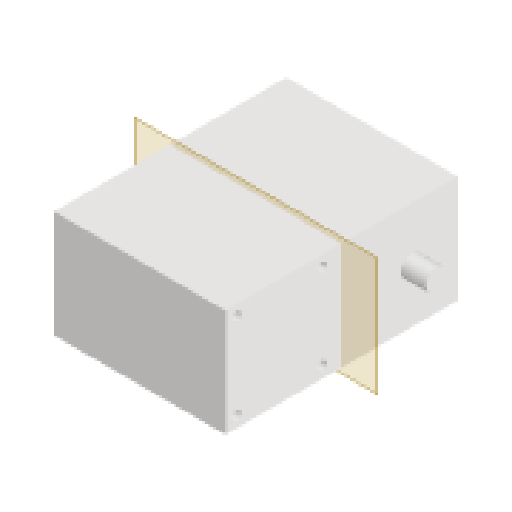
# Autodesk Inventor part: рдс150
Saved by Autodesk Inventor 2023.2 (Build 272271030, 271C)
## iProperties
Created: 2025-05-06
Part Number: рдс150
Material: Типовые
Document SubType Name: Modeling
Designer: Олег Коноваленко
Density: 1 g/cm^3
Appearance: По умолчанию
Author: Олег Коноваленко
Autodesk Inventor part; units mm, degrees
ref_plane "YZ Plane" through (0, 0, 0) normal (1, 0, 0) x (0, 1, 0)
ref_plane "XZ Plane" through (0, 0, 0) normal (0, 1, 0) x (-1, 0, 0)
ref_plane "XY Plane" through (0, 0, 0) normal (0, 0, 1) x (1, 0, 0)
sketch "Эскиз1" plane through (0, 0, 0) normal (0, 1, 0) x (-1, 0, 0)
  line L0 (24, -32.5) -> (-24, -32.5)
  line L1 (-24, -32.5) -> (-24, 32.5)
  line L2 (-24, 32.5) -> (24, 32.5)
  line L3 (24, 32.5) -> (24, -32.5)
  line L4 (24, -32.5) -> (-24, 32.5) construction
  line L5 (-24, -32.5) -> (24, 32.5) construction
  line L6 (-33.6, 0) -> (33.6, 0) construction
  line L7 (0, -45.5) -> (0, 45.5) projected
  point P0 (0, 0)
  point P1 (0, 0)
  point P2 (0, 0)
  dimension "d0" = 65
  dimension "d1" = 48
  constraints: 12 end point, 4 midpoint, 2 parallel, 1 horizontal, 1 perpendicular
  measures "d0" distance of L0.end L1.end
  measures "d1" distance of L0.start L0.end
extrude "Выдавливание1" add sketch "Эскиз1" along normal mid plane 30
sketch "Эскиз2" plane through (24, -15, -32.5) normal (1, 0, 0) x (0, 0, -1)
  circle A0 centre (-62, 27) radius 1.35
  circle A1 centre (-38, 27) radius 1.35
  circle A2 centre (-38, 3) radius 1.35
  circle A3 centre (-62, 3) radius 1.35
  line L0 (-62, 27) -> (-38, 27) construction
  line L1 (-38, 27) -> (-38, 3) construction
  line L2 (-38, 3) -> (-62, 3) construction
  line L3 (-62, 27) -> (-62, 3) construction
  line L4 (-65, 30) -> (0, 30) projected
  line L5 (-65, 0) -> (-65, 30) projected
  point P0 (-32.5, 15)
  dimension "d4" = 2.7
  dimension "d9" = 24
  dimension "d10" = 3
  dimension "d11" = 3
  constraints: 8 end point, 4 centre point, 3 equal radius, 3 perpendicular, 1 horizontal, 1 parallel
  measures "d4" diameter of A0
  measures "d9" distance of L0.start L0.end
  measures "d10" distance from line of L4 L0.start
  measures "d11" distance from line of L5 L0.start
extrude "Выдавливание2" cut sketch "Эскиз2" against normal up to surface (24 mm away)
sketch "Эскиз3" plane through (-24, -15, 32.5) normal (-1, 0, 0) x (0, 0, 1)
  line L0 (-15, 27) -> (-3, 27)
  line L1 (-3, 27) -> (-3, 3)
  line L2 (-3, 3) -> (-15, 3)
  circle A0 centre (-3, 15) radius 1.35
  circle A1 centre (-15, 27) radius 1.35
  circle A2 centre (-15, 3) radius 1.35
  line L3 (-65, 30) -> (0, 30) projected
  line L4 (0, 30) -> (0, 0) projected
  point P0 (-32.5, 15)
  dimension "d14" = 24
  dimension "d15" = 12
  dimension "d17" = 2.7
  dimension "d18" = 3
  dimension "d19" = 3
  constraints: 6 end point, 3 centre point, 3 coincident, 2 equal radius, 2 perpendicular, 1 horizontal, 1 midpoint, 1 parallel
  measures "d14" distance of L0.end L1.end
  measures "d15" distance of L0.start L0.end
  measures "d17" diameter of A0
  measures "d18" distance between parallel lines of L3 L0
  measures "d19" distance between parallel lines of L4 L1
extrude "Выдавливание3" cut sketch "Эскиз3" against normal up to surface (24 mm away)
sketch "Эскиз4" plane through (-24, -15, 32.5) normal (-1, 0, 0) x (0, 0, 1)
  circle A0 centre (-52, 15) radius 3
  line L0 (-78, 15) -> (13, 15) projected
  line L1 (-65, 0) -> (-65, 30) projected
  point P0 (-32.5, 15)
  dimension "d22" = 6
  dimension "d23" = 13
  constraints: 1 centre point, 1 point on line
  measures "d22" diameter of A0
  measures "d23" distance from line of L1 A0.centre
extrude "Выдавливание4" add sketch "Эскиз4" along normal blind 7
mirror "Зеркальное отражение1" about plane through (0, 0, 0) normal (1, 0, 0) of "Выдавливание4"
